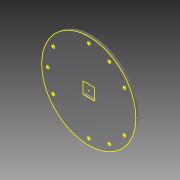
# Autodesk Inventor part: top top plate
Saved by Autodesk Inventor 2015 (Build 190159000, 159)
## iProperties
Created: 2015-10-18
Part Number: top top plate
Material: Polycarbonate, Clear
Document SubType Name: Modeling
Designer: Brian
Density: 1.2 g/cm^3
Appearance: Polycarbonate - Clear
Mass: 29.1774 g
Surface Area: 175.885 cm^2
Volume: 24.3145 cm^3
Author: Brian
Autodesk Inventor part; units mm, degrees
ref_plane "YZ Plane" through (0, 0, 0) normal (1, 0, 0) x (0, 1, 0)
ref_plane "XZ Plane" through (0, 0, 0) normal (0, 1, 0) x (-1, 0, 0)
ref_plane "XY Plane" through (0, 0, 0) normal (0, 0, 1) x (1, 0, 0)
sketch "Sketch1" plane through (0, 0, 0) normal (0, 1, 0) x (-1, 0, 0)
  circle A0 centre (0, 0) radius 51.5
  line L0 (-6.4, 6.4) -> (6.4, 6.4)
  line L1 (6.4, 6.4) -> (6.4, -6.4)
  line L2 (6.4, -6.4) -> (-6.4, -6.4)
  line L3 (-6.4, -6.4) -> (-6.4, 6.4)
  line L4 (-6.4, 6.4) -> (6.4, -6.4) construction
  line L5 (6.4, 6.4) -> (-6.4, -6.4) construction
  dimension "d0" = 103
  dimension "d1" = 12.8
  dimension "d2" = 12.8
  constraints: 12 end point, 2 midpoint, 2 parallel, 1 centre point, 1 coincident, 1 horizontal, 1 perpendicular
  measures "d0" diameter of A0
  measures "d1" distance of L2.end L0.start
  measures "d2" distance of L1.end L2.end
extrude "Extrusion1" add sketch "Sketch1" along normal blind 3
sketch "Sketch2" plane through (0, 3, 0) normal (0, 1, 0) x (1, 0, 0)
  line L0 (-6.4, -6.4) -> (-6.4, 6.4) construction
  line L1 (-6.4, 6.4) -> (6.4, 6.4) construction
  line L2 (6.4, 6.4) -> (6.4, -6.4) construction
  line L3 (6.4, -6.4) -> (-6.4, -6.4) construction
  circle A0 centre (0, 0) radius 51.5 construction
  line L4 (6.4, 0) -> (51.5, 0) construction
  circle A1 centre (0, 0) radius 51.5 construction
  line L5 (0, 0) -> (-25.75, 44.6003) construction
  line L6 (0, 0) -> (-25.75, -44.6003) construction
  circle A2 centre (0, 0) radius 45 construction
  line L7 (0, 0) -> (0, -51.5) construction
  line L8 (0, 0) -> (44.6003, -25.75) construction
  line L9 (0, 0) -> (25.75, -44.6003) construction
  line L10 (0, 0) -> (25.75, 44.6003) construction
  line L11 (44.6003, 25.75) -> (0, 0) construction
  line L12 (0, 0) -> (0, 51.5) construction
  line L13 (0, 0) -> (-44.6003, -25.75) construction
  line L14 (0, 0) -> (-51.5, 0) construction
  line L15 (0, 0) -> (-44.6003, 25.75) construction
  circle A3 centre (38.9711, -22.5) radius 1.5
  circle A4 centre (22.5, -38.9711) radius 1.5
  circle A5 centre (0, -45) radius 1.5
  circle A6 centre (-38.9711, -22.5) radius 1.5
  circle A7 centre (-45, 0) radius 1.5
  circle A8 centre (-38.9711, 22.5) radius 1.5
  circle A9 centre (22.5, 38.9711) radius 1.5
  circle A10 centre (38.9711, 22.5) radius 1.5
  circle A11 centre (0, 45) radius 1.5
  dimension "d7" = 90
  dimension "d5" = 120
  dimension "d6" = 120
  dimension "d8" = 30
  dimension "d9" = 30
  dimension "d10" = 30
  dimension "d11" = 30
  dimension "d12" = 30
  dimension "d13" = 30
  dimension "d14" = 30
  dimension "d15" = 30
  dimension "d16" = 3
  dimension "d17" = 3
  dimension "d18" = 3
  dimension "d19" = 3
  dimension "d20" = 3
  dimension "d21" = 3
  dimension "d22" = 3
  dimension "d23" = 3
  dimension "d24" = 3
  constraints: 24 end point, 9 centre point, 9 point on line, 1 coincident, 1 horizontal, 1 midpoint, 1 perpendicular, 37 other
  measures "d5" angle of L4 L6
  measures "d6" angle of L4 L5
  measures "d8" angle of L8 L4
  measures "d9" angle of L7 L9
  measures "d10" angle of L6 L7
  measures "d11" angle of L13 L6
  measures "d12" angle of L13 L14
  measures "d13" angle of L14 L15
  measures "d14" angle of L5 L12
  measures "d15" angle of L10 L12
  measures "d16" diameter of A3
  measures "d17" diameter of A4
  measures "d18" diameter of A5
  measures "d19" diameter of A6
  measures "d20" diameter of A7
  measures "d21" diameter of A8
  measures "d22" diameter of A9
  measures "d23" diameter of A10
  measures "d24" diameter of A11
extrude "Extrusion2" cut sketch "Sketch2" against normal blind 3
sketch "Sketch3" plane through (0, 0, 0) normal (0, -1, 0) x (1, 0, 0)
  circle A0 centre (38.9711, -22.5) radius 1.5 projected
  circle A1 centre (-38.9711, -22.5) radius 1.5 projected
  circle A2 centre (-38.9711, 22.5) radius 1.5 projected
  circle A3 centre (22.5, 38.9711) radius 1.5 projected
  circle A4 centre (38.9711, 22.5) radius 1.5 projected
  circle A5 centre (0, 45) radius 1.5 projected
  circle A6 centre (-45, 0) radius 1.5 projected
  circle A7 centre (22.5, -38.9711) radius 1.5 projected
  circle A8 centre (0, -45) radius 1.5 projected
  line L0 (-6.4, -6.4) -> (-6.4, 6.4) projected
  line L1 (-6.4, 6.4) -> (6.4, 6.4) projected
  line L2 (6.4, 6.4) -> (6.4, -6.4) projected
  line L3 (6.4, -6.4) -> (-6.4, -6.4) projected
  circle A9 centre (0, 0) radius 51.5 projected
equation "\"d2\" = d1"
equation "\"d9\" = d8"
equation "\"d10\" = d8"
equation "\"d11\" = d8"
equation "\"d12\" = d8"
equation "\"d13\" = d8"
equation "\"d14\" = d8"
equation "\"d15\" = d8"
equation "\"d17\" = d16"
equation "\"d18\" = d16"
equation "\"d19\" = d16"
equation "\"d20\" = d16"
equation "\"d21\" = d16"
equation "\"d22\" = d16"
equation "\"d23\" = d16"
equation "\"d24\" = d16"
body "Solid1"
